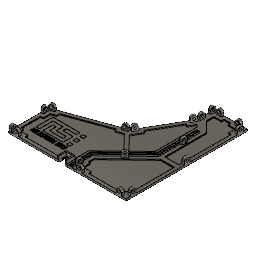
smmb_side-left (Autodesk Fusion 360 design; units mm, degrees)
Autodesk Fusion 360 part; units mm, degrees
(part 1 of 2)
sketch "Sketch1" plane through (0, 0, 0) normal (0, 0, 1) x (1, 0, 0)
  line L0 (0, 0) -> (36.5, 63.2199)
  line L1 (0, 0) -> (72, 0) construction
  line L2 (0, 0) -> (-88.801, -32.3209)
  line L3 (0, 0) -> (95, 0) construction
  line L4 (-88.801, -32.3209) -> (-88.801, -92.3209)
  line L5 (36.5, 63.2199) -> (36.5, 88.2199)
  line L6 (36.5, 88.2199) -> (86.5, 88.2199)
  line L7 (86.5, 88.2199) -> (86.5, -92.3209)
  line L8 (-88.801, -92.3209) -> (-85.7851, -92.3209)
  line L9 (-85.7851, -92.3209) -> (86.5, -92.3209)
  line L10 (-1.0261, 1.2228) -> (-90.301, -31.2706)
  line L11 (-90.301, -31.2706) -> (-90.301, -93.8209)
  line L12 (-90.301, -93.8209) -> (-85.7851, -93.8209)
  line L13 (-85.7851, -93.8209) -> (88, -93.8209)
  line L14 (88, 89.7199) -> (88, -93.8209)
  line L15 (35, 89.7199) -> (88, 89.7199)
  line L16 (35, 63.6218) -> (35, 89.7199)
  line L17 (-1.0261, 1.2228) -> (35, 63.6218)
  line L18 (-88.801, -92.3209) -> (-88.801, -93.8209)
  line L19 (86.5, -92.3209) -> (86.5, -93.8209)
  line L20 (-89.7879, -32.6801) -> (-88.801, -32.3209)
  line L21 (-90.301, -31.2706) -> (-89.7879, -32.6801)
  line L22 (-88.801, -32.3209) -> (-90.301, -32.3209)
  line L23 (-1.0261, 1.2228) -> (0.273, 0.4728)
  line L24 (-1.0261, 1.2228) -> (-0.513, -0.1867)
  line L25 (35, 63.6218) -> (36.299, 62.8718)
  line L26 (35, 63.6218) -> (36.5, 63.6218)
  line L27 (36.5, 88.2199) -> (36.5, 89.7199)
  line L28 (86.5, 88.2199) -> (86.5, 89.7199)
  line L29 (36.299, 62.8718) -> (31.299, 54.2115)
  line L30 (31.299, 54.2115) -> (44.2894, 46.7115)
  line L31 (44.2894, 46.7115) -> (18.2894, 1.6782)
  line L32 (18.2894, 1.6782) -> (5.299, 9.1782)
  line L33 (54.5, -92.3209) -> (53, -92.3209)
  line L34 (53, -92.3209) -> (53, 47.6791)
  line L35 (53, 47.6791) -> (54.5, 47.6791)
  line L36 (54.5, 47.6791) -> (54.5, -92.3209)
  line L37 (53, 47.6791) -> (53, -12.3209)
  line L38 (53, -12.3209) -> (2.6462, -60.947)
  line L39 (53, -12.3209) -> (123.075, -12.3209) construction
  line L40 (2.6462, -60.947) -> (2.6462, -92.3209)
  line L41 (54.5, 47.6791) -> (54.5, -12.9576)
  line L42 (54.5, -12.9576) -> (4.1462, -61.5837)
  line L43 (4.1462, -61.5837) -> (4.1462, -92.3209)
  line L44 (2.273, 3.9369) -> (8.9375, 0.0891)
  line L45 (36.299, 62.8718) -> (34.299, 59.4077)
  line L46 (-0.513, -0.1867) -> (-4.2718, -1.5548)
  line L47 (-0.513, -0.1867) -> (3.487, -0.1867) construction
  line L48 (-89.7879, -32.6801) -> (-84.1498, -30.628)
  line L49 (-88.801, -32.3209) -> (-88.801, -40.3209)
  line L50 (-88.801, -93.8209) -> (-88.801, -87.8209)
  line L51 (36.5, 63.6218) -> (36.5, 67.6218)
  line L52 (36.5, 89.7199) -> (36.5, 83.7199)
  line L53 (36.5, 88.2199) -> (47.5, 88.2199)
  line L54 (86.5, 88.2199) -> (75.5, 88.2199)
  line L55 (86.5, 89.7199) -> (86.5, 77.7199)
  line L56 (86.5, -93.8209) -> (86.5, -81.8209)
  line L57 (88, -2.0505) -> (86.5, -2.0505)
  line L58 (-88.801, -93.8209) -> (-77.801, -93.8209)
  line L59 (86.5, -93.8209) -> (75.5, -93.8209)
  line L60 (86.5, -93.8209) -> (16.5, -93.8209)
  line L61 (52.7, 47.6791) -> (52.7, -12.1936)
  line L62 (52.7, -12.1936) -> (2.3462, -60.8196)
  line L63 (2.3462, -60.8196) -> (2.3462, -92.3209)
  line L64 (54.8, 47.6791) -> (54.8, -13.085)
  line L65 (54.8, -13.085) -> (4.4462, -61.711)
  line L66 (4.4462, -61.711) -> (4.4462, -92.3209)
  line L67 (51.7, 47.6791) -> (51.7, -11.7691)
  line L68 (51.7, -11.7691) -> (1.3462, -60.3952)
  line L69 (1.3462, -60.3952) -> (1.3462, -92.3209)
  line L70 (55.8, 47.6791) -> (55.8, -13.5094)
  line L71 (55.8, -13.5094) -> (5.4462, -62.1355)
  line L72 (5.4462, -62.1355) -> (5.4462, -92.3209)
  line L73 (51.7, 47.6791) -> (55.8, 47.6791)
  line L74 (2.6462, -60.947) -> (4.1462, -62.447) construction
  line L75 (2.6462, -60.947) -> (4.7675, -60.947) construction
  line L76 (4.1462, -62.447) -> (2.6462, -62.447) construction
  line L77 (4.4462, -61.711) -> (3.1958, -60.4162) construction
  dimension "d3" = 60
  dimension "d4" = 73
  dimension "d5" = 160
  dimension "d6" = 94.5
  dimension "d7" = 60
  dimension "d8" = 25
  dimension "d9" = 90
  dimension "d10" = 50
  dimension "d11" = -1.5
  dimension "d12" = 71.0521
  dimension "d13" = 95.5044
  dimension "d15" = 61.5
  dimension "d16" = 10
  dimension "d17" = 15
  dimension "d18" = 52
  dimension "d19" = 140
  dimension "d20" = 1.5
  dimension "d21" = 32
  dimension "d22" = 60
  dimension "d23" = 136
  dimension "d24" = 70
  dimension "d25" = -1.5
  dimension "d26" = 4
  dimension "d34" = 4
  dimension "d39" = 160
  dimension "d40" = 4
  dimension "d41" = 6
  dimension "d51" = 8
  dimension "d57" = 6
  dimension "d61" = 4
  dimension "d62" = 6
  dimension "d71" = 11
  dimension "d72" = 11
  dimension "d81" = 12
  dimension "d82" = 12
  dimension "d91" = 183.5408
  dimension "d92" = 91.7704
  dimension "d96" = 11
  dimension "d97" = 11
  dimension "d98" = 70
  dimension "d109" = 0.3
  dimension "d110" = -1.8
  dimension "d111" = 1.3
  dimension "d112" = -2.8
  dimension "d154" = 26.0981
  dimension "d155" = 175.301
  dimension "d157" = 45
  dimension "d158" = 29.8739
  dimension "d160" = 0.7641
  constraint horizontal L1
  constraint coincident L0.start L1.start
  constraint horizontal L3
  constraint vertical L4
  constraint vertical L5
  constraint perpendicular L6 L7
  constraint perpendicular L4 L8
  constraint perpendicular L7 L9
  constraint coincident L12 L18.end
  constraint perpendicular L12 L18
  constraint coincident L13 L19.end
  constraint perpendicular L13 L19
  constraint parallel L2 L20
  constraint perpendicular L20 L21
  constraint coincident L11 L22.end
  constraint perpendicular L11 L22
  constraint coincident L0 L23.end
  constraint perpendicular L0 L23
  constraint coincident L2 L24.end
  constraint perpendicular L2 L24
  constraint coincident L0 L25.end
  constraint perpendicular L0 L25
  constraint coincident L5 L26.end
  constraint perpendicular L5 L26
  constraint coincident L15 L27.end
  constraint perpendicular L15 L27
  constraint coincident L15 L28.end
  constraint perpendicular L15 L28
  constraint coincident L0 L29.end
  constraint perpendicular L29 L30
  constraint perpendicular L25 L31
  constraint coincident L0 L32.end
  constraint perpendicular L0 L32
  constraint horizontal L33
  constraint vertical L34
  constraint horizontal L35
  constraint vertical L36
  constraint coincident L9 L33.start
  constraint perpendicular L3 L37
  constraint horizontal L39
  constraint coincident L9 L40.end
  constraint perpendicular L9 L40
  constraint coincident L0 L44.start
  constraint perpendicular L0 L44
  constraint perpendicular L25 L45
  constraint horizontal L47
  constraint perpendicular L21 L48
  constraint vertical L49
  constraint perpendicular L22 L49
  constraint perpendicular L8 L50
  constraint vertical L51
  constraint perpendicular L6 L52
  constraint perpendicular L52 L53
  constraint perpendicular L7 L54
  constraint perpendicular L15 L55
  constraint perpendicular L9 L56
  constraint coincident L14 L57.start
  constraint coincident L7 L57.end
  constraint perpendicular L7 L57
  constraint perpendicular L50 L58
  constraint perpendicular L19 L59
  constraint perpendicular L19 L60
  constraint perpendicular L70 L73
  constraint horizontal L75
  constraint coincident L43 L74.end
  constraint coincident L40 L76.end
  constraint perpendicular L40 L76
  constraint coincident L38 L77.end
  constraint perpendicular L38 L77
  measures "d3" angle of L0 L1
  measures "d4" distance of L0.start L0.end
  measures "d5" angle of L2 L3
  measures "d6" distance of L0.start L2.end
  measures "d7" distance of L2.end L4.end
  measures "d8" distance of L0.end L5.end
  measures "d9" angle of L5 L6
  measures "d10" distance of L5.end L6.end
  measures "d15" distance of L2.end L12
  measures "d16" distance of L25.end L29.end
  measures "d17" distance of L29.end L30.end
  measures "d18" distance of L30.end L31.end
  measures "d19" distance of L33.start L35.end
  measures "d20" distance of L33.start L33.end
  measures "d21" distance of L7 L36
  measures "d22" distance of L34.end L37.end
  measures "d23" angle of L38 L39
  measures "d24" distance of L37.end L38.end
  measures "d26" distance of L23 L44
  measures "d34" distance of L25.end L45.end
  measures "d39" angle of L46 L47
  measures "d40" distance of L24.end L46.end
  measures "d41" distance of L20.start L48.end
  measures "d51" distance of L2.end L49.end
  measures "d57" distance of L18.end L50.end
  measures "d61" distance of L26.end L51.end
  measures "d62" distance of L27.end L52.end
  measures "d71" distance of L5.end L53.end
  measures "d72" distance of L6.end L54.end
  measures "d81" distance of L28.end L55.end
  measures "d82" distance of L19.end L56.end
  measures "d91" distance of L13.end L14.start
  measures "d92" distance of L15 L57
  measures "d96" distance of L18.end L58.end
  measures "d97" distance of L19.end L59.end
  measures "d98" distance of L19.end L60.end
  measures "d154" distance of L15 L26
  measures "d155" distance of L4 L7
  measures "d157" angle of L74 L75
  measures "d158" distance of L9 L76
  measures "d160" distance of L38.end L77.end
extrude "Extrude1" add sketch "Sketch1" along normal blind 3 contours L0 L2 L4 L5 L6 L7 L8 L9 L29 L30 L31 L32 L35 L36 L45 L46 L48 L49 L50 L51 L52 L53 L54 L55 L56 L67 L68 L69 L70 L71 L73 | L0 L30 L31 L32 | L9 L61 L62 L63 L67 L68 L69 L73 | L9 L34 L37 L38 L40 L61 L62 L63 L73 | L9 L34 L38 L40 L42 L43 | L9 L34 L42 L43 L65 L66 | L9 L33 L34 L36 L71 | L9 L34 L65 L66 L71 L72 | L34 L35 L36 L37 L41 L42 L73 | L9 L34 L71 L72 | L34 L36 L65 L71 | L36 L64 L65 L70 L71 L73 | L34 L36 L42 L65 | L36 L41 L64 L65 L73
sketch "Sketch2" plane through (0, 0, 0) normal (-0.866025, 0.5, 0) x (-0.5, -0.866025, 0)
  line L0 (-73, 0) -> (0, 0)
  line L1 (0, 0) -> (0, 3)
  line L2 (0, 3) -> (-73, 3)
  line L3 (-73, 3) -> (-73, 0)
  line L4 (-4.546, 0) -> (-4.546, 7)
  circle A0 centre (-4.546, 7) radius 2.05
  circle A1 centre (-4.546, 7) radius 4.05
  line L5 (-0.496, 7) -> (-0.496, 3)
  line L6 (-8.596, 7) -> (-8.596, 3)
  line L7 (-68.5413, 0) -> (-68.5413, 7)
  circle A2 centre (-68.5413, 7) radius 2.05
  circle A3 centre (-68.5413, 7) radius 4.05
  line L8 (-64.4913, 7) -> (-64.4913, 3)
  line L9 (-94.6506, 3) -> (-73, 3)
  line L10 (-72.5913, 7) -> (-72.5913, 3)
  point P0 (-4.546, 0)
  point P1 (-68.5413, 0)
  dimension "d29" = 7
  dimension "d30" = 4.1
  dimension "d31" = 8.1
  dimension "d36" = 7
  dimension "d37" = 4.1
  dimension "d38" = 8.1
  constraint vertical L4
  constraint coincident P0 L4.start
  constraint coincident L4.end A0.centre
  constraint concentric A0 A1
  constraint coincident A1 L5.start
  constraint coincident L2 L5.end
  constraint perpendicular L2 L5
  constraint tangent A1 L5
  constraint coincident A1 L6.start
  constraint coincident L2 L6.end
  constraint tangent A1 L6
  constraint perpendicular L2 L6
  constraint vertical L7
  constraint coincident P1 L7.start
  constraint coincident L7.end A2.centre
  constraint concentric A2 A3
  constraint coincident A3 L8.start
  constraint coincident L2 L8.end
  constraint perpendicular L2 L8
  constraint tangent A3 L8
  constraint coincident A3 L10.start
  constraint coincident L9 L10.end
  constraint tangent A3 L10
  constraint perpendicular L2 L10
  measures "d29" distance of P0 L4.end
  measures "d30" diameter of A0
  measures "d31" diameter of A1
  measures "d36" distance of P1 L7.end
  measures "d37" diameter of A2
  measures "d38" diameter of A3
extrude "Extrude2" add sketch "Sketch2" against normal blind 4 contours L2 A3 L10 | L2 A3 | L2 A3 L8 | L2 A1 | L2 A1 L6 | L2 A1 L5
sketch "Sketch3" plane through (0, 0, 0) normal (-0.34202, 0.939693, 0) x (-0.939693, -0.34202, 0)
  line L0 (0, 0) -> (94.5, 0)
  line L1 (94.5, 0) -> (94.5, 3)
  line L2 (94.5, 3) -> (0, 3)
  line L3 (0, 3) -> (0, 0)
  line L4 (4.546, 0) -> (4.546, 7)
  line L5 (89.5503, 0) -> (89.5503, 7)
  circle A0 centre (4.546, 7) radius 2.05
  circle A1 centre (4.546, 7) radius 4.05
  line L6 (8.596, 7) -> (8.596, 2.9796)
  line L7 (0.496, 7) -> (0.496, 3)
  circle A2 centre (89.5503, 7) radius 2.05
  circle A3 centre (89.5503, 7) radius 4.05
  line L8 (85.5003, 7) -> (85.5003, 3)
  line L9 (93.6003, 7) -> (93.6003, 3)
  point P0 (4.546, 0)
  point P1 (89.5503, 0)
  dimension "d42" = 7
  dimension "d43" = 7
  dimension "d44" = 4.1
  dimension "d45" = 8.1
  dimension "d46" = 4.1
  dimension "d47" = 8.1
  constraint vertical L4
  constraint coincident P0 L4.start
  constraint coincident P1 L5.start
  constraint perpendicular L0 L5
  constraint coincident L4.end A0.centre
  constraint concentric A0 A1
  constraint vertical L6
  constraint coincident A1 L6.start
  constraint tangent A1 L6
  constraint vertical L7
  constraint coincident A1 L7.start
  constraint coincident L2 L7.end
  constraint tangent A1 L7
  constraint coincident L5.end A2.centre
  constraint concentric A2 A3
  constraint coincident A3 L8.start
  constraint coincident L2 L8.end
  constraint perpendicular L2 L8
  constraint tangent A3 L8
  constraint coincident A3 L9.start
  constraint coincident L2 L9.end
  constraint tangent A3 L9
  constraint perpendicular L2 L9
  measures "d42" distance of P0 L4.end
  measures "d43" distance of P1 L5.end
  measures "d44" diameter of A0
  measures "d45" diameter of A1
  measures "d46" diameter of A2
  measures "d47" diameter of A3
extrude "Extrude3" add sketch "Sketch3" against normal blind 4 contours L2 A1 L7 | L2 A1 | L2 A1 L6 | L2 A3 | L2 A3 L8 | L2 A3 L9
sketch "Sketch4" plane through (0, 0, 3) normal (0, 0, 1) x (-1, 0, 0)
  line L0 (80.344, 29.2428) -> (78.9759, 33.0016)
  line L1 (78.9759, 33.0016) -> (86.5874, 35.772)
  line L2 (86.5874, 35.772) -> (87.9555, 32.0132)
  line L3 (87.9555, 32.0132) -> (88.801, 32.3209)
  line L4 (88.801, 32.3209) -> (88.801, 92.3209)
  line L5 (88.801, 92.3209) -> (-86.5, 92.3209)
  line L6 (-86.5, 92.3209) -> (-86.5, -88.2199)
  line L7 (-86.5, -88.2199) -> (-36.5, -88.2199)
  line L8 (-36.5, -88.2199) -> (-36.5, -63.2199)
  line L9 (-36.5, -63.2199) -> (-36.2957, -62.8659)
  line L10 (-36.2957, -62.8659) -> (-39.7598, -60.8659)
  line L11 (-39.7598, -60.8659) -> (-35.7098, -53.8511)
  line L12 (-35.7098, -53.8511) -> (-32.2457, -55.8511)
  line L13 (-32.2457, -55.8511) -> (-4.298, -7.4443)
  line L14 (-4.298, -7.4443) -> (-7.7621, -5.4443)
  line L15 (-7.7621, -5.4443) -> (-3.7121, 1.5705)
  line L16 (-3.7121, 1.5705) -> (-0.248, -0.4295)
  line L17 (-0.248, -0.4295) -> (0, 0)
  line L18 (0, 0) -> (0.466, 0.1696)
  line L19 (0.466, 0.1696) -> (-0.902, 3.9284)
  line L20 (-0.902, 3.9284) -> (6.7095, 6.6988)
  line L21 (6.7095, 6.6988) -> (8.0776, 2.94)
  line L22 (8.0776, 2.94) -> (80.344, 29.2428)
  line L23 (-36.5, -68.0615) -> (-47.3532, -61.7954)
  line L24 (-47.3532, -61.7954) -> (0.4629, 21.0245)
  line L25 (0.4629, 21.0245) -> (22.0469, 8.0244)
  line L26 (22.0469, 8.0244) -> (-36.5, -68.0615)
  constraint coincident L8 L23.start
  constraint parallel L12 L23
  constraint perpendicular L23 L24
  constraint coincident L22 L25.end
sketch "Sketch5" plane through (-88.801, 0, 0) normal (-1, 0, 0) x (0, -1, 0)
  line L0 (32.3209, 0) -> (92.3209, 0)
  line L1 (92.3209, 0) -> (92.3209, 3)
  line L2 (92.3209, 3) -> (32.3209, 3)
  line L3 (32.3209, 3) -> (32.3209, 0)
  line L4 (40.3209, 0) -> (40.3209, 7)
  circle A0 centre (40.3209, 7) radius 2.05
  circle A1 centre (40.3209, 7) radius 4.05
  line L5 (44.3709, 7) -> (44.3709, 3)
  line L6 (36.2709, 7) -> (36.2709, 3)
  line L7 (87.8209, 0) -> (87.8209, 7)
  circle A2 centre (87.8209, 7) radius 2.05
  circle A3 centre (87.8209, 7) radius 4.05
  line L8 (91.8709, 7) -> (91.8709, 3)
  line L9 (83.7709, 7) -> (83.7709, 3)
  point P0 (40.3209, 0)
  point P1 (87.8209, 0)
  dimension "d52" = 7
  dimension "d53" = 4.1
  dimension "d54" = 8.1
  dimension "d58" = 7
  dimension "d59" = 4.1
  dimension "d60" = 8.1
  constraint vertical L4
  constraint coincident P0 L4.start
  constraint coincident L4.end A0.centre
  constraint concentric A0 A1
  constraint vertical L5
  constraint coincident A1 L5.start
  constraint coincident L2 L5.end
  constraint tangent A1 L5
  constraint coincident A1 L6.start
  constraint coincident L2 L6.end
  constraint perpendicular L2 L6
  constraint tangent A1 L6
  constraint coincident P1 L7.start
  constraint perpendicular L0 L7
  constraint coincident L7.end A2.centre
  constraint concentric A2 A3
  constraint coincident A3 L8.start
  constraint coincident L2 L8.end
  constraint coincident A3 L9.start
  constraint coincident L2 L9.end
  constraint tangent A3 L8
  constraint tangent A3 L9
  constraint perpendicular L2 L8
  constraint perpendicular L2 L9
  measures "d52" distance of P0 L4.end
  measures "d53" diameter of A0
  measures "d54" diameter of A1
  measures "d58" distance of P1 L7.end
  measures "d59" diameter of A2
  measures "d60" diameter of A3
extrude "Extrude4" add sketch "Sketch5" against normal blind 4 contours L2 A1 L6 | L2 A1 | L2 A1 L5 | L2 A3 | L2 A3 L9 | L2 A3 L8
sketch "Sketch6" plane through (36.5, 0, 0) normal (-1, 0, 0) x (0, -1, 0)
  line L0 (-88.2199, 0) -> (-63.2199, 0)
  line L1 (-63.2199, 0) -> (-63.2199, 3)
  line L2 (-63.2199, 3) -> (-88.2199, 3)
  line L3 (-88.2199, 3) -> (-88.2199, 0)
  line L4 (-67.6218, 0) -> (-67.6218, 7)
  line L5 (-83.7199, 0) -> (-83.7199, 7)
  circle A0 centre (-67.6218, 7) radius 2.05
  circle A1 centre (-67.6218, 7) radius 4.05
  line L6 (-63.5718, 7) -> (-63.5718, 3)
  line L7 (-71.6718, 7) -> (-71.6718, 3)
  circle A2 centre (-83.7199, 7) radius 2.05
  circle A3 centre (-83.7199, 7) radius 4.05
  line L8 (-79.6699, 7) -> (-79.6699, 3)
  line L9 (-87.7699, 7) -> (-87.7699, 3)
  point P0 (-67.6218, 0)
  point P1 (-83.7199, 0)
  dimension "d63" = 7
  dimension "d64" = 7
  dimension "d65" = 4.1
  dimension "d66" = 8.1
  dimension "d67" = 4.1
  dimension "d68" = 8.1
  constraint vertical L4
  constraint coincident P0 L4.start
  constraint vertical L5
  constraint coincident P1 L5.start
  constraint coincident L4.end A0.centre
  constraint concentric A0 A1
  constraint coincident A1 L6.start
  constraint coincident L2 L6.end
  constraint coincident A1 L7.start
  constraint coincident L2 L7.end
  constraint coincident L5.end A2.centre
  constraint concentric A2 A3
  constraint coincident A3 L8.start
  constraint coincident L2 L8.end
  constraint coincident A3 L9.start
  constraint coincident L2 L9.end
  constraint tangent A1 L6
  constraint tangent A1 L7
  constraint tangent A3 L8
  constraint tangent A3 L9
  constraint perpendicular L2 L6
  constraint perpendicular L2 L7
  constraint perpendicular L2 L8
  constraint perpendicular L2 L9
  measures "d63" distance of P0 L4.end
  measures "d64" distance of P1 L5.end
  measures "d65" diameter of A2
  measures "d66" diameter of A3
  measures "d67" diameter of A0
  measures "d68" diameter of A1
extrude "Extrude5" add sketch "Sketch6" against normal blind 4 contours L2 A3 L9 | L2 A3 | L2 A3 L8 | L2 A1 | L2 A1 L7 | L2 A1 L6
sketch "Sketch7" plane through (0, 88.2199, 0) normal (0, 1, 0) x (-1, 0, 0)
  line L0 (-86.5, 0) -> (-36.5, 0)
  line L1 (-36.5, 0) -> (-36.5, 3)
  line L2 (-36.5, 3) -> (-86.5, 3)
  line L3 (-86.5, 3) -> (-86.5, 0)
  line L4 (-75.5, 0) -> (-75.5, 7)
  line L5 (-47.5, 0) -> (-47.5, 7)
  circle A0 centre (-75.5, 7) radius 2.05
  circle A1 centre (-75.5, 7) radius 4.05
  line L6 (-71.45, 7) -> (-71.45, 3)
  line L7 (-79.55, 7) -> (-79.55, 3)
  circle A2 centre (-47.5, 7) radius 2.05
  circle A3 centre (-47.5, 7) radius 4.05
  line L8 (-51.55, 7) -> (-51.55, 3)
  line L9 (-43.45, 7) -> (-43.45, 3)
  point P0 (-75.5, 0)
  point P1 (-47.5, 0)
  point P2 (-36.5, 7)
  dimension "d73" = 7
  dimension "d74" = 7
  dimension "d75" = 4.1
  dimension "d76" = 8.1
  dimension "d77" = 4.1
  dimension "d78" = 8.1
  constraint coincident P0 L4.start
  constraint perpendicular L0 L4
  constraint coincident P1 L5.start
  constraint perpendicular L0 L5
  constraint coincident L4.end A0.centre
  constraint concentric A0 A1
  constraint coincident A1 L6.start
  constraint coincident L2 L6.end
  constraint coincident A1 L7.start
  constraint coincident L2 L7.end
  constraint tangent A1 L6
  constraint tangent A1 L7
  constraint perpendicular L2 L6
  constraint perpendicular L2 L7
  constraint coincident L5.end A2.centre
  constraint concentric A2 A3
  constraint coincident A3 L8.start
  constraint coincident L2 L8.end
  constraint perpendicular L2 L8
  constraint tangent A3 L8
  constraint coincident A3 L9.start
  constraint coincident L2 L9.end
  constraint tangent A3 L9
  constraint perpendicular L2 L9
  measures "d73" distance of P0 L4.end
  measures "d74" distance of P1 L5.end
  measures "d75" diameter of A0
  measures "d76" diameter of A1
  measures "d77" diameter of A2
  measures "d78" diameter of A3
extrude "Extrude6" add sketch "Sketch7" against normal blind 4 contours L2 A1 L7 | L2 A1 | L2 A1 L6 | L2 A3 | L2 A3 L8 | L2 A3 L9
sketch "Sketch8" plane through (86.5, 0, 0) normal (1, 0, 0) x (0, 1, 0)
  line L0 (-92.3209, 0) -> (88.2199, 0)
  line L1 (88.2199, 0) -> (88.2199, 3)
  line L2 (88.2199, 3) -> (-92.3209, 3)
  line L3 (-92.3209, 3) -> (-92.3209, 0)
  line L4 (77.7199, 0) -> (77.7199, 7)
  circle A0 centre (77.7199, 7) radius 2.05
  circle A1 centre (77.7199, 7) radius 4.05
  line L5 (73.6699, 7) -> (73.6699, 3)
  line L6 (81.7699, 7) -> (81.7699, 3)
  line L7 (-81.8209, 0) -> (-81.8209, 7)
  circle A2 centre (-81.8209, 7) radius 2.05
  circle A3 centre (-81.8209, 7) radius 4.05
  line L8 (-77.7709, 7) -> (-77.7709, 3)
  line L9 (-85.8709, 7) -> (-85.8709, 3)
  line L10 (-1.5548, 0) -> (-1.5548, 7)
  circle A4 centre (-1.5548, 7) radius 2.05
  circle A5 centre (-1.5548, 7) radius 4.05
  line L11 (2.4952, 7) -> (2.4952, 3)
  line L12 (-5.6048, 7) -> (-5.6048, 3)
  point P0 (77.7199, 0)
  point P1 (-81.8209, 0)
  point P2 (-1.5548, 0)
  dimension "d83" = 7
  dimension "d84" = 4.1
  dimension "d85" = 8.1
  dimension "d86" = 7
  dimension "d87" = 4.1
  dimension "d88" = 8.1
  dimension "d93" = 7
  dimension "d94" = 4.1
  dimension "d95" = 8.1
  constraint coincident P0 L4.start
  constraint perpendicular L0 L4
  constraint coincident L4.end A0.centre
  constraint concentric A0 A1
  constraint coincident A1 L5.start
  constraint coincident L2 L5.end
  constraint coincident A1 L6.start
  constraint coincident L2 L6.end
  constraint perpendicular L2 L6
  constraint perpendicular L2 L5
  constraint tangent A1 L6
  constraint tangent A1 L5
  constraint coincident P1 L7.start
  constraint perpendicular L0 L7
  constraint coincident L7.end A2.centre
  constraint concentric A2 A3
  constraint coincident A3 L8.start
  constraint coincident L2 L8.end
  constraint coincident A3 L9.start
  constraint coincident L2 L9.end
  constraint perpendicular L2 L8
  constraint perpendicular L2 L9
  constraint tangent A3 L8
  constraint tangent A3 L9
  constraint vertical L10
  constraint coincident P2 L10.start
  constraint coincident L10.end A4.centre
  constraint concentric A4 A5
  constraint coincident A5 L11.start
  constraint coincident L2 L11.end
  constraint coincident A5 L12.start
  constraint coincident L2 L12.end
  constraint perpendicular L2 L11
  constraint perpendicular L2 L12
  constraint tangent A5 L11
  constraint tangent A5 L12
  measures "d83" distance of P0 L4.end
  measures "d84" diameter of A0
  measures "d85" diameter of A1
  measures "d86" distance of P1 L7.end
  measures "d87" diameter of A2
  measures "d88" diameter of A3
  measures "d93" distance of P2 L10.end
  measures "d94" diameter of A4
  measures "d95" diameter of A5
extrude "Extrude7" add sketch "Sketch8" against normal blind 4 contours L2 A3 L9 | L2 A3 | L2 A3 L8 | L2 A5 | L2 A5 L12 | L2 A5 L11 | L2 A1 | L2 A1 L5 | L2 A1 L6
sketch "Sketch9" plane through (0, -92.3209, 0) normal (0, -1, 0) x (1, 0, 0)
  line L0 (-88.801, 0) -> (86.5, 0)
  line L1 (86.5, 0) -> (86.5, 3)
  line L2 (86.5, 3) -> (-88.801, 3)
  line L3 (-88.801, 3) -> (-88.801, 0)
  line L4 (16.5, 0) -> (16.5, 7)
  line L5 (-77.801, 0) -> (-77.801, 7)
  line L6 (75.5, 0) -> (75.5, 7)
  circle A0 centre (75.5, 7) radius 2.05
  circle A1 centre (75.5, 7) radius 4.05
  line L7 (79.55, 7) -> (79.55, 3)
  line L8 (71.45, 7) -> (71.45, 3)
  circle A2 centre (16.5, 7) radius 2.05
  circle A3 centre (16.5, 7) radius 4.05
  line L9 (20.55, 7) -> (20.55, 3)
  line L10 (12.45, 7) -> (12.45, 3)
  circle A4 centre (-77.801, 7) radius 2.05
  circle A5 centre (-77.801, 7) radius 4.05
  line L11 (-73.751, 7) -> (-73.751, 3)
  line L12 (-81.851, 7) -> (-81.851, 3)
  point P0 (16.5, 0)
  point P1 (-77.801, 0)
  point P2 (75.5, 0)
  point P3 (77.55, 7)
  point P4 (79.55, 7)
  point P5 (79.55, 3)
  point P6 (71.45, 7)
  point P7 (71.45, 3)
  dimension "d99" = 7
  dimension "d100" = 7
  dimension "d101" = 7
  dimension "d102" = 4.1
  dimension "d103" = 8.1
  dimension "d104" = 4.1
  dimension "d105" = 8.1
  constraint coincident P0 L4.start
  constraint perpendicular L0 L4
  constraint coincident P1 L5.start
  constraint perpendicular L0 L5
  constraint coincident P2 L6.start
  constraint perpendicular L2 L6
  constraint coincident L6.end A0.centre
  constraint coincident A0 P3
  constraint concentric A0 A1
  constraint coincident A1 P4
  constraint coincident P4 L7.start
  constraint coincident P5 L7.end
  constraint coincident P6 L8.start
  constraint coincident P7 L8.end
  constraint coincident L4.end A2.centre
  constraint concentric A2 A3
  constraint coincident A3 L9.start
  constraint coincident L2 L9.end
  constraint coincident A3 L10.start
  constraint coincident L2 L10.end
  constraint tangent A3 L9
  constraint tangent A3 L10
  constraint perpendicular L2 L9
  constraint perpendicular L2 L10
  constraint coincident L5.end A4.centre
  constraint concentric A4 A5
  constraint coincident A5 L11.start
  constraint coincident L2 L11.end
  constraint coincident A5 L12.start
  constraint coincident L2 L12.end
  constraint tangent A5 L12
  constraint tangent A5 L11
  constraint perpendicular L2 L11
  constraint perpendicular L2 L12
  measures "d99" distance of P0 L4.end
  measures "d100" distance of P1 L5.end
  measures "d101" distance of P2 L6.end
  measures "d102" diameter of A2
  measures "d103" diameter of A3
  measures "d104" diameter of A4
  measures "d105" diameter of A5
extrude "Extrude8" add sketch "Sketch9" against normal blind 4 contours L2 A5 L12 | L2 A5 | L2 A5 L11 | L2 A3 | L2 A3 L10 | L2 A3 L9 | L2 A1 | L2 A1 L8 | L2 A1 L7
extrude "Extrude9" add sketch "Sketch1" along normal blind 5 contours L9 L61 L62 L63 L67 L68 L69 L73 | L9 L34 L65 L66 L71 L72 | L34 L36 L65 L71 | L36 L64 L65 L70 L71 L73
sketch "Sketch10" plane through (4.4462, 0, 0) normal (-1, 0, 0) x (0, -1, 0)
  line L0 (61.711, 3) -> (92.3209, 3)
  line L1 (92.3209, 3) -> (92.3209, 5)
  line L2 (92.3209, 5) -> (61.711, 5)
  line L3 (61.711, 5) -> (61.711, 3)
  line L4 (32.3209, 0) -> (92.3209, 0)
  line L5 (81.8209, 0) -> (81.8209, 7)
  line L6 (92.3209, 0) -> (92.3209, 3)
  circle A0 centre (81.8209, 7) radius 2.05
  circle A1 centre (81.8209, 7) radius 4.05
  line L7 (77.7709, 7) -> (77.7709, 3)
  line L8 (85.8709, 7) -> (85.8709, 3)
  line L9 (77.7709, 3) -> (77.7709, 0)
  line L10 (85.8709, 3) -> (85.8709, 0)
  point P0 (77.7709, 7)
  point P1 (77.7709, 3)
  point P2 (85.8709, 7)
  point P3 (85.8709, 3)
  dimension "d115" = 7
  dimension "d116" = 10.5
  dimension "d125" = 4.1
  constraint coincident L4 L5.start
  constraint perpendicular L4 L5
  constraint coincident L5.end A0.centre
  constraint concentric A0 A1
  constraint coincident P0 L7.start
  constraint coincident P1 L7.end
  constraint coincident P2 L8.start
  constraint coincident P3 L8.end
  constraint tangent A1 L8
  constraint coincident L4 L9.end
  constraint perpendicular L4 L9
  constraint coincident L4 L10.end
  constraint perpendicular L4 L10
  measures "d115" distance of L5.start L5.end
  measures "d116" distance of L5 L6
  measures "d125" diameter of A0
sketch "Sketch11" plane through (32.9822, -34.1541, 0) normal (-0.694658, 0.71934, 0) x (-0.71934, -0.694658, 0)
  line L0 (-30.3302, 3) -> (39.6698, 3)
  line L1 (39.6698, 3) -> (39.6698, 5)
  line L2 (39.6698, 5) -> (-30.3302, 5)
  line L3 (-30.3302, 5) -> (-30.3302, 3)
  line L4 (39.6698, 3) -> (4.6698, 3)
  circle A0 centre (4.6698, 7) radius 2.05
  circle A1 centre (4.6698, 7) radius 4.05
  line L5 (0.6198, 7) -> (0.6198, 5)
  line L6 (8.7198, 7) -> (8.7198, 5)
  line L7 (0, 0) -> (86.33, 0)
  line L8 (4.6698, 7) -> (4.6698, 0)
  line L9 (0.6198, 5) -> (0.6198, 0)
  line L10 (8.7198, 5) -> (8.7198, 0)
  dimension "d119" = 4.1
  dimension "d120" = 8.1
  dimension "d126" = 7
  dimension "d156" = 35
  constraint coincident L0.end L1.start
  constraint midpoint L0 L4.end
  constraint concentric A0 A1
  constraint coincident A1 L5.start
  constraint coincident L2 L5.end
  constraint tangent A1 L5
  constraint perpendicular L2 L5
  constraint coincident A1 L6.start
  constraint coincident L2 L6.end
  constraint tangent A1 L6
  constraint perpendicular L2 L6
  constraint coincident A0.centre A1.centre
  constraint coincident L7 L8.end
  constraint perpendicular L4 L8
  constraint coincident L7 L9.end
  constraint perpendicular L7 L9
  constraint coincident L7 L10.end
  constraint perpendicular L7 L10
  measures "d119" diameter of A0
  measures "d120" diameter of A1
  measures "d126" distance of A0.centre L8.end
  measures "d156" distance of L1 L8
sketch "Sketch12" plane through (54.8, 0, 0) normal (-1, 0, 0) x (0, -1, 0)
  line L0 (-47.6791, 3) -> (13.085, 3)
  line L1 (13.085, 3) -> (13.085, 5)
  line L2 (13.085, 5) -> (-47.6791, 5)
  line L3 (-47.6791, 5) -> (-47.6791, 3)
  line L4 (-47.6791, 3) -> (-22.6791, 3)
  line L5 (-63.2199, 0) -> (0, 0)
  line L6 (-22.6791, 0) -> (-22.6791, 7)
  circle A0 centre (-22.6791, 7) radius 2.05
  circle A1 centre (-22.6791, 7) radius 4.05
  line L7 (-18.6291, 7) -> (-18.6291, 0)
  line L8 (-26.7291, 7) -> (-26.7291, 0)
  dimension "d121" = 25
  dimension "d128" = 7
  dimension "d129" = 4.1
  dimension "d130" = 8.1
  constraint coincident L0.start L3.end
  constraint perpendicular L3 L4
  constraint coincident L5 L6.start
  constraint perpendicular L5 L6
  constraint coincident L6.end A0.centre
  constraint concentric A0 A1
  constraint coincident A1 L7.start
  constraint coincident L5 L7.end
  constraint tangent A1 L7
  constraint perpendicular L5 L7
  constraint coincident A1 L8.start
  constraint coincident L5 L8.end
  constraint tangent A1 L8
  constraint perpendicular L5 L8
  measures "d121" distance of L0.start L4.end
  measures "d128" distance of L6.start L6.end
  measures "d129" diameter of A0
  measures "d130" diameter of A1
extrude "Extrude10" add sketch "Sketch12" against normal blind 4 contours L0 L2 L4 A1 L8 | L0 L4 L5 L6 A1 L8 | L0 L2 L4 L6 A0 A1 | L0 L4 L6 A1 | L2 A1 L8 | L0 L2 L6 A0 A1 | L0 L6 A1 | L2 A0 A1 | L0 L5 L6 A1 L7 | L0 L2 A1 L7 | L2 A1 L7
extrude "Extrude11" add sketch "Sketch11" against normal blind 4 contours L0 L2 A1 L9 | L0 A1 L7 L8 L9 | L0 L2 A0 A1 L8 | L0 A1 L8 | L2 A1 L5 | L0 L2 L4 A0 A1 L8 | L0 L4 A1 L8 | L2 A0 A1 | L0 L4 A1 L7 L8 L10 | L0 L2 L4 A1 L10 | L2 A1 L6
extrude "Extrude12" add sketch "Sketch10" against normal blind 4 contours L0 L2 A1 L7 | L0 L4 L5 A1 L9 | L0 L2 L5 A0 A1 | L0 L5 A1 | L2 A1 L7 | L0 L2 L5 A0 A1 | L0 L5 A1 | L2 A0 A1 | L0 L4 L5 A1 L10 | L0 L2 A1 L8 | L2 A1 L8
sketch "Sketch13" plane through (0, 0, 3) normal (0, 0, 1) x (-1, 0, 0)
  line L0 (-5.4462, 77.7709) -> (-8.4462, 77.7709)
  line L1 (-8.4462, 77.7709) -> (-8.4462, 85.8709)
  line L2 (-8.4462, 85.8709) -> (-5.4462, 85.8709)
  line L3 (-5.4462, 85.8709) -> (-5.4462, 92.3209)
  line L4 (-5.4462, 92.3209) -> (-12.45, 92.3209)
  line L5 (-12.45, 92.3209) -> (-12.45, 88.3209)
  line L6 (-12.45, 88.3209) -> (-20.55, 88.3209)
  line L7 (-20.55, 88.3209) -> (-20.55, 92.3209)
  line L8 (-20.55, 92.3209) -> (-71.45, 92.3209)
  line L9 (-71.45, 92.3209) -> (-71.45, 88.3209)
  line L10 (-71.45, 88.3209) -> (-79.55, 88.3209)
  line L11 (-79.55, 88.3209) -> (-79.55, 92.3209)
  line L12 (-79.55, 92.3209) -> (-86.5, 92.3209)
  line L13 (-86.5, 92.3209) -> (-86.5, 85.8709)
  line L14 (-86.5, 85.8709) -> (-82.5, 85.8709)
  line L15 (-82.5, 85.8709) -> (-82.5, 77.7709)
  line L16 (-82.5, 77.7709) -> (-86.5, 77.7709)
  line L17 (-86.5, 77.7709) -> (-86.5, 5.6048)
  line L18 (-86.5, 5.6048) -> (-82.5, 5.6048)
  line L19 (-82.5, 5.6048) -> (-82.5, -2.4952)
  line L20 (-82.5, -2.4952) -> (-86.5, -2.4952)
  line L21 (-86.5, -2.4952) -> (-86.5, -73.6699)
  line L22 (-86.5, -73.6699) -> (-82.5, -73.6699)
  line L23 (-82.5, -73.6699) -> (-82.5, -81.7699)
  line L24 (-82.5, -81.7699) -> (-86.5, -81.7699)
  line L25 (-86.5, -81.7699) -> (-86.5, -88.2199)
  line L26 (-86.5, -88.2199) -> (-79.55, -88.2199)
  line L27 (-79.55, -88.2199) -> (-79.55, -84.2199)
  line L28 (-79.55, -84.2199) -> (-71.45, -84.2199)
  line L29 (-71.45, -84.2199) -> (-71.45, -88.2199)
  line L30 (-71.45, -88.2199) -> (-51.55, -88.2199)
  line L31 (-51.55, -88.2199) -> (-51.55, -84.2199)
  line L32 (-51.55, -84.2199) -> (-43.45, -84.2199)
  line L33 (-43.45, -84.2199) -> (-43.45, -88.2199)
  line L34 (-43.45, -88.2199) -> (-36.5, -88.2199)
  line L35 (-36.5, -88.2199) -> (-36.5, -87.7699)
  line L36 (-36.5, -87.7699) -> (-40.5, -87.7699)
  line L37 (-40.5, -87.7699) -> (-40.5, -79.6699)
  line L38 (-40.5, -79.6699) -> (-36.5, -79.6699)
  line L39 (-36.5, -79.6699) -> (-36.5, -71.6718)
  line L40 (-36.5, -71.6718) -> (-40.5, -71.6718)
  line L41 (-40.5, -71.6718) -> (-40.5, -63.5718)
  line L42 (-40.5, -63.5718) -> (-36.5, -63.5718)
  line L43 (-36.5, -63.5718) -> (-36.5, -63.2199)
  line L44 (-36.5, -63.2199) -> (-36.2957, -62.8659)
  line L45 (-36.2957, -62.8659) -> (-39.7598, -60.8659)
  line L46 (-39.7598, -60.8659) -> (-35.7098, -53.8511)
  line L47 (-35.7098, -53.8511) -> (-32.2457, -55.8511)
  line L48 (-32.2457, -55.8511) -> (-4.298, -7.4443)
  line L49 (-4.298, -7.4443) -> (-7.7621, -5.4443)
  line L50 (-7.7621, -5.4443) -> (-3.7121, 1.5705)
  line L51 (-3.7121, 1.5705) -> (-0.248, -0.4295)
  line L52 (-0.248, -0.4295) -> (0, 0)
  line L53 (0, 0) -> (0.466, 0.1696)
  line L54 (0.466, 0.1696) -> (-0.902, 3.9284)
  line L55 (-0.902, 3.9284) -> (6.7095, 6.6988)
  line L56 (6.7095, 6.6988) -> (8.0776, 2.94)
  line L57 (8.0776, 2.94) -> (80.344, 29.2428)
  line L58 (80.344, 29.2428) -> (78.9759, 33.0016)
  line L59 (78.9759, 33.0016) -> (86.5874, 35.772)
  line L60 (86.5874, 35.772) -> (87.9555, 32.0132)
  line L61 (87.9555, 32.0132) -> (88.801, 32.3209)
  line L62 (88.801, 32.3209) -> (88.801, 36.2709)
  line L63 (88.801, 36.2709) -> (84.801, 36.2709)
  line L64 (84.801, 36.2709) -> (84.801, 44.3709)
  line L65 (84.801, 44.3709) -> (88.801, 44.3709)
  line L66 (88.801, 44.3709) -> (88.801, 83.7709)
  line L67 (88.801, 83.7709) -> (84.801, 83.7709)
  line L68 (84.801, 83.7709) -> (84.801, 91.8709)
  line L69 (84.801, 91.8709) -> (88.801, 91.8709)
  line L70 (88.801, 91.8709) -> (88.801, 92.3209)
  line L71 (88.801, 92.3209) -> (81.851, 92.3209)
  line L72 (81.851, 92.3209) -> (81.851, 88.3209)
  line L73 (81.851, 88.3209) -> (73.751, 88.3209)
  line L74 (73.751, 88.3209) -> (73.751, 92.3209)
  line L75 (73.751, 92.3209) -> (-1.3462, 92.3209)
  line L76 (-1.3462, 92.3209) -> (-1.3462, 60.3952)
  line L77 (-1.3462, 60.3952) -> (-51.7, 11.7691)
  line L78 (-51.7, 11.7691) -> (-51.7, -47.6791)
  line L79 (-51.7, -47.6791) -> (-52.7, -47.6791)
  line L80 (-52.7, -47.6791) -> (-52.7, 12.1936)
  line L81 (-52.7, 12.1936) -> (-2.3462, 60.8196)
  line L82 (-2.3462, 60.8196) -> (-2.3462, 92.3209)
  line L83 (-2.3462, 92.3209) -> (-4.4462, 92.3209)
  line L84 (-4.4462, 92.3209) -> (-4.4462, 61.711)
  line L85 (-4.4462, 61.711) -> (-54.8, 13.085)
  line L86 (-54.8, 13.085) -> (-54.8, -47.6791)
  line L87 (-54.8, -47.6791) -> (-55.8, -47.6791)
  line L88 (-55.8, -47.6791) -> (-55.8, -26.7291)
  line L89 (-55.8, -26.7291) -> (-58.8, -26.7291)
  line L90 (-58.8, -26.7291) -> (-58.8, -18.6291)
  line L91 (-58.8, -18.6291) -> (-55.8, -18.6291)
  line L92 (-55.8, -18.6291) -> (-55.8, 13.5094)
  line L93 (-55.8, 13.5094) -> (-33.2311, 35.304)
  line L94 (-33.2311, 35.304) -> (-35.3151, 37.462)
  line L95 (-35.3151, 37.462) -> (-29.4884, 43.0887)
  line L96 (-29.4884, 43.0887) -> (-27.4044, 40.9307)
  line L97 (-27.4044, 40.9307) -> (-5.4462, 62.1355)
  line L98 (-5.4462, 62.1355) -> (-5.4462, 77.7709)
  line L99 (3.6538, 58.2728) -> (-46.7, 9.6467)
  line L100 (-46.7, 9.6467) -> (-46.7, -52.6791)
  line L101 (-46.7, -52.6791) -> (-49.8, -52.6791)
  line L102 (-49.8, -52.6791) -> (-57.7, -52.6791)
  line L103 (-57.7, -52.6791) -> (-60.8, -52.6791)
  line L104 (-60.8, -52.6791) -> (-60.8, 15.6318)
  line L105 (-60.8, 15.6318) -> (-10.4462, 64.2579)
  line L106 (-10.4462, 64.2579) -> (-10.4462, 72.7709)
  line L107 (-10.4462, 72.7709) -> (-13.4462, 72.7709)
  line L108 (-13.4462, 72.7709) -> (-13.4462, 83.3209)
  line L109 (-13.4462, 83.3209) -> (-25.55, 83.3209)
  line L110 (-25.55, 83.3209) -> (-25.55, 87.3209)
  line L111 (-25.55, 87.3209) -> (-66.45, 87.3209)
  line L112 (-66.45, 87.3209) -> (-66.45, 83.3209)
  line L113 (-66.45, 83.3209) -> (-77.5, 83.3209)
  line L114 (-77.5, 83.3209) -> (-77.5, 72.7709)
  line L115 (-77.5, 72.7709) -> (-81.5, 72.7709)
  line L116 (-81.5, 72.7709) -> (-81.5, -68.6699)
  line L117 (-81.5, -68.6699) -> (-77.5, -68.6699)
  line L118 (-77.5, -68.6699) -> (-77.5, -79.2199)
  line L119 (-77.5, -79.2199) -> (-66.45, -79.2199)
  line L120 (-66.45, -79.2199) -> (-66.45, -83.2199)
  line L121 (-66.45, -83.2199) -> (-56.55, -83.2199)
  line L122 (-56.55, -83.2199) -> (-56.55, -79.2199)
  line L123 (-56.55, -79.2199) -> (-45.5, -79.2199)
  line L124 (-45.5, -79.2199) -> (-45.5, -76.6718)
  line L125 (-45.5, -76.6718) -> (-45.5, -74.6699)
  line L126 (-45.5, -60.8083) -> (-37.5399, -47.021)
  line L127 (-45.5, -74.6699) -> (-45.5, -60.8083)
  line L128 (-37.5399, -47.021) -> (-34.0758, -49.021)
  line L129 (-34.0758, -49.021) -> (-11.1281, -9.2744)
  line L130 (-11.1281, -9.2744) -> (-14.5922, -7.2744)
  line L131 (-14.5922, -7.2744) -> (-6.1564, 7.3369)
  line L132 (-6.1564, 7.3369) -> (9.6978, 13.1073)
  line L133 (9.6978, 13.1073) -> (11.0659, 9.3486)
  line L134 (11.0659, 9.3486) -> (73.9354, 32.2312)
  line L135 (73.9354, 32.2312) -> (72.5674, 35.99)
  line L136 (72.5674, 35.99) -> (79.801, 38.6228)
  line L137 (79.801, 38.6228) -> (79.801, 49.3709)
  line L138 (79.801, 49.3709) -> (83.801, 49.3709)
  line L139 (83.801, 49.3709) -> (83.801, 78.7709)
  line L140 (83.801, 78.7709) -> (79.801, 78.7709)
  line L141 (79.801, 78.7709) -> (79.801, 83.3209)
  line L142 (79.801, 83.3209) -> (68.751, 83.3209)
  line L143 (68.751, 83.3209) -> (68.751, 87.3209)
  line L144 (68.751, 87.3209) -> (3.6538, 87.3209)
  line L145 (3.6538, 87.3209) -> (3.6538, 58.2728)
  line L146 (-60.8, -52.6791) -> (-45.5, -67.9791)
  line L147 (-60.8, -52.6791) -> (-39.1625, -52.6791) construction
  line L148 (-46.7, -52.6791) -> (-42.9637, -56.4154)
  line L149 (-60.8, 15.6318) -> (-81.5, 15.6318)
  line L150 (-60.8, 9.3067) -> (-81.5, 9.3067)
  line L151 (-6.1564, 7.3369) -> (-26.8749, 28.7916)
  line L152 (-0.7443, 9.3067) -> (-23.0901, 32.4465)
  dimension "d162" = 45
  constraint parallel L77 L99
  constraint parallel L78 L100
  constraint parallel L79 L101
  constraint parallel L79 L102
  constraint parallel L87 L103
  constraint parallel L88 L104
  constraint parallel L92 L104
  constraint parallel L93 L105
  constraint parallel L97 L105
  constraint parallel L98 L106
  constraint parallel L0 L107
  constraint parallel L1 L108
  constraint parallel L6 L109
  constraint parallel L7 L110
  constraint parallel L8 L111
  constraint parallel L9 L112
  constraint parallel L10 L113
  constraint parallel L15 L114
  constraint parallel L16 L115
  constraint parallel L17 L116
  constraint parallel L21 L116
  constraint parallel L22 L117
  constraint parallel L23 L118
  constraint parallel L28 L119
  constraint parallel L29 L120
  constraint parallel L30 L121
  constraint parallel L31 L122
  constraint parallel L32 L123
  constraint parallel L37 L124
  constraint parallel L37 L125
  constraint parallel L41 L127
  constraint parallel L46 L126
  constraint parallel L47 L128
  constraint parallel L48 L129
  constraint parallel L49 L130
  constraint parallel L50 L131
  constraint parallel L55 L132
  constraint parallel L56 L133
  constraint parallel L57 L134
  constraint parallel L58 L135
  constraint parallel L59 L136
  constraint parallel L64 L137
  constraint parallel L65 L138
  constraint parallel L66 L139
  constraint parallel L67 L140
  constraint parallel L68 L141
  constraint parallel L73 L142
  constraint parallel L74 L143
  constraint parallel L75 L144
  constraint parallel L76 L145
  constraint horizontal L147
  constraint coincident L127 L146.end
  constraint coincident L126 L148.end
  constraint parallel L146 L148
  constraint coincident L116 L149.end
  constraint perpendicular L116 L149
  constraint coincident L104 L150.start
  constraint coincident L116 L150.end
  constraint perpendicular L116 L150
  constraint coincident L99 L151.end
  constraint perpendicular L99 L151
  constraint coincident L132 L152.start
  constraint coincident L99 L152.end
  constraint perpendicular L99 L152
  measures "d162" angle of L146 L147
sketch "Sketch14" plane through (0, 0, 3) normal (0, 0, 1) x (-1, 0, 0)
  line L0 (-5.4462, 77.7709) -> (-8.4462, 77.7709)
  line L1 (-8.4462, 77.7709) -> (-8.4462, 85.8709)
  line L2 (-8.4462, 85.8709) -> (-5.4462, 85.8709)
  line L3 (-5.4462, 85.8709) -> (-5.4462, 92.3209)
  line L4 (-5.4462, 92.3209) -> (-12.45, 92.3209)
  line L5 (-12.45, 92.3209) -> (-12.45, 88.3209)
  line L6 (-12.45, 88.3209) -> (-20.55, 88.3209)
  line L7 (-20.55, 88.3209) -> (-20.55, 92.3209)
  line L8 (-20.55, 92.3209) -> (-71.45, 92.3209)
  line L9 (-71.45, 92.3209) -> (-71.45, 88.3209)
  line L10 (-71.45, 88.3209) -> (-79.55, 88.3209)
  line L11 (-79.55, 88.3209) -> (-79.55, 92.3209)
  line L12 (-79.55, 92.3209) -> (-86.5, 92.3209)
  line L13 (-86.5, 92.3209) -> (-86.5, 85.8709)
  line L14 (-86.5, 85.8709) -> (-82.5, 85.8709)
  line L15 (-82.5, 85.8709) -> (-82.5, 77.7709)
  line L16 (-82.5, 77.7709) -> (-86.5, 77.7709)
  line L17 (-86.5, 77.7709) -> (-86.5, 5.6048)
  line L18 (-86.5, 5.6048) -> (-82.5, 5.6048)
  line L19 (-82.5, 5.6048) -> (-82.5, -2.4952)
  line L20 (-82.5, -2.4952) -> (-86.5, -2.4952)
  line L21 (-86.5, -2.4952) -> (-86.5, -73.6699)
  line L22 (-86.5, -73.6699) -> (-82.5, -73.6699)
  line L23 (-82.5, -73.6699) -> (-82.5, -81.7699)
  line L24 (-82.5, -81.7699) -> (-86.5, -81.7699)
  line L25 (-86.5, -81.7699) -> (-86.5, -88.2199)
  line L26 (-86.5, -88.2199) -> (-79.55, -88.2199)
  line L27 (-79.55, -88.2199) -> (-79.55, -84.2199)
  line L28 (-79.55, -84.2199) -> (-71.45, -84.2199)
  line L29 (-71.45, -84.2199) -> (-71.45, -88.2199)
  line L30 (-71.45, -88.2199) -> (-51.55, -88.2199)
  line L31 (-51.55, -88.2199) -> (-51.55, -84.2199)
  line L32 (-51.55, -84.2199) -> (-43.45, -84.2199)
  line L33 (-43.45, -84.2199) -> (-43.45, -88.2199)
  line L34 (-43.45, -88.2199) -> (-36.5, -88.2199)
  line L35 (-36.5, -88.2199) -> (-36.5, -87.7699)
  line L36 (-36.5, -87.7699) -> (-40.5, -87.7699)
  line L37 (-40.5, -87.7699) -> (-40.5, -79.6699)
  line L38 (-40.5, -79.6699) -> (-36.5, -79.6699)
  line L39 (-36.5, -79.6699) -> (-36.5, -71.6718)
  line L40 (-36.5, -71.6718) -> (-40.5, -71.6718)
  line L41 (-40.5, -71.6718) -> (-40.5, -63.5718)
  line L42 (-40.5, -63.5718) -> (-36.5, -63.5718)
  line L43 (-36.5, -63.5718) -> (-36.5, -63.2199)
  line L44 (-36.5, -63.2199) -> (-36.2957, -62.8659)
  line L45 (-36.2957, -62.8659) -> (-39.7598, -60.8659)
  line L46 (-39.7598, -60.8659) -> (-35.7098, -53.8511)
  line L47 (-35.7098, -53.8511) -> (-32.2457, -55.8511)
  line L48 (-32.2457, -55.8511) -> (-4.298, -7.4443)
  line L49 (-4.298, -7.4443) -> (-7.7621, -5.4443)
  line L50 (-7.7621, -5.4443) -> (-3.7121, 1.5705)
  line L51 (-3.7121, 1.5705) -> (-0.248, -0.4295)
  line L52 (-0.248, -0.4295) -> (0, 0)
  line L53 (0, 0) -> (0.466, 0.1696)
  line L54 (0.466, 0.1696) -> (-0.902, 3.9284)
  line L55 (-0.902, 3.9284) -> (6.7095, 6.6988)
  line L56 (6.7095, 6.6988) -> (8.0776, 2.94)
  line L57 (8.0776, 2.94) -> (80.344, 29.2428)
  line L58 (80.344, 29.2428) -> (78.9759, 33.0016)
  line L59 (78.9759, 33.0016) -> (86.5874, 35.772)
  line L60 (86.5874, 35.772) -> (87.9555, 32.0132)
  line L61 (87.9555, 32.0132) -> (88.801, 32.3209)
  line L62 (88.801, 32.3209) -> (88.801, 36.2709)
  line L63 (88.801, 36.2709) -> (84.801, 36.2709)
  line L64 (84.801, 36.2709) -> (84.801, 44.3709)
  line L65 (84.801, 44.3709) -> (88.801, 44.3709)
  line L66 (88.801, 44.3709) -> (88.801, 83.7709)
  line L67 (88.801, 83.7709) -> (84.801, 83.7709)
  line L68 (84.801, 83.7709) -> (84.801, 91.8709)
  line L69 (84.801, 91.8709) -> (88.801, 91.8709)
  line L70 (88.801, 91.8709) -> (88.801, 92.3209)
  line L71 (88.801, 92.3209) -> (81.851, 92.3209)
  line L72 (81.851, 92.3209) -> (81.851, 88.3209)
  line L73 (81.851, 88.3209) -> (73.751, 88.3209)
  line L74 (73.751, 88.3209) -> (73.751, 92.3209)
  line L75 (73.751, 92.3209) -> (-1.3462, 92.3209)
  line L76 (-1.3462, 92.3209) -> (-1.3462, 60.3952)
  line L77 (-1.3462, 60.3952) -> (-51.7, 11.7691)
  line L78 (-51.7, 11.7691) -> (-51.7, -47.6791)
  line L79 (-51.7, -47.6791) -> (-52.7, -47.6791)
  line L80 (-52.7, -47.6791) -> (-52.7, 12.1936)
  line L81 (-52.7, 12.1936) -> (-2.3462, 60.8196)
  line L82 (-2.3462, 60.8196) -> (-2.3462, 92.3209)
  line L83 (-2.3462, 92.3209) -> (-4.4462, 92.3209)
  line L84 (-4.4462, 92.3209) -> (-4.4462, 61.711)
  line L85 (-4.4462, 61.711) -> (-54.8, 13.085)
  line L86 (-54.8, 13.085) -> (-54.8, -47.6791)
  line L87 (-54.8, -47.6791) -> (-55.8, -47.6791)
  line L88 (-55.8, -47.6791) -> (-55.8, -26.7291)
  line L89 (-55.8, -26.7291) -> (-58.8, -26.7291)
  line L90 (-58.8, -26.7291) -> (-58.8, -18.6291)
  line L91 (-58.8, -18.6291) -> (-55.8, -18.6291)
  line L92 (-55.8, -18.6291) -> (-55.8, 13.5094)
  line L93 (-55.8, 13.5094) -> (-33.2311, 35.304)
  line L94 (-33.2311, 35.304) -> (-35.3151, 37.462)
  line L95 (-35.3151, 37.462) -> (-29.4884, 43.0887)
  line L96 (-29.4884, 43.0887) -> (-27.4044, 40.9307)
  line L97 (-27.4044, 40.9307) -> (-5.4462, 62.1355)
  line L98 (-5.4462, 62.1355) -> (-5.4462, 77.7709)
  line L99 (4.801, 92.3209) -> (13.801, 92.3209)
  line L100 (13.801, 92.3209) -> (13.801, 81.3209)
  line L101 (13.801, 81.3209) -> (4.801, 81.3209)
  line L102 (4.801, 81.3209) -> (4.801, 92.3209)
  line L103 (2.801, 79.3209) -> (2.801, 94.3209)
  line L104 (2.801, 94.3209) -> (15.801, 94.3209)
  line L105 (15.801, 94.3209) -> (15.801, 79.3209)
  line L106 (15.801, 79.3209) -> (2.801, 79.3209)
  dimension "d139" = 9
  dimension "d140" = 11
  dimension "d141" = 75
  dimension "d142" = -2
  constraint horizontal L99
  constraint vertical L100
  constraint horizontal L101
  constraint vertical L102
  constraint coincident L75 L99.start
  measures "d139" distance of L99.start L99.end
  measures "d140" distance of L99.start L101.end
  measures "d141" distance of L66 L100
extrude "Extrude14" cut sketch "Sketch14" against normal blind 3 contours L75 L99 L100 L101 L102
extrude "Extrude15" add sketch "Sketch14" along normal blind 5 contours L75 L100 L101 L102 L103 L105 L106